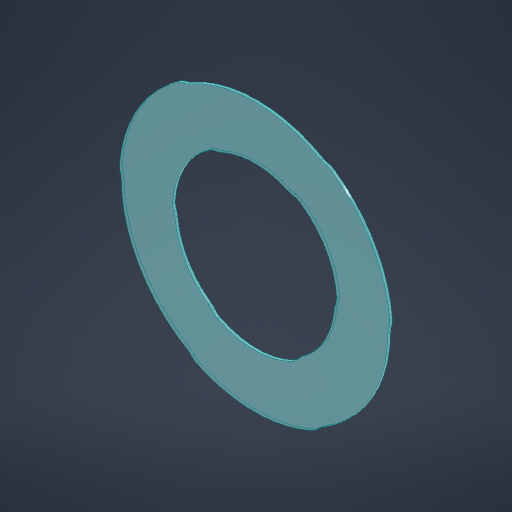
# Autodesk Inventor part: Lid_B
Saved by Autodesk Inventor 2026.1 (Build 301233020, 233B)
## iProperties
Created: 2023-08-16
Part Number: Lid_B
Material: PMMA Plastic
Document SubType Name: Modeling
Designer: Joshua Harper
Density: 1.188 g/cm^3
Appearance: Polycarbonate - Clear
Author: Joshua Harper
Autodesk Inventor part; units mm, degrees
ref_plane "YZ Plane" through (0, 0, 0) normal (1, 0, 0) x (0, 1, 0)
ref_plane "XZ Plane" through (0, 0, 0) normal (0, 1, 0) x (-1, 0, 0)
ref_plane "XY Plane" through (0, 0, 0) normal (0, 0, 1) x (1, 0, 0)
sketch "Sketch1" plane through (0, 0, 0) normal (0, 0, 1) x (1, 0, 0)
  circle A0 centre (0, 0) radius 106
  circle A1 centre (0, 0) radius 62.5
  dimension "d0" = 212
  dimension "d1" = 125
  constraints: 2 centre point, 2 coincident
  measures "d0" diameter of A0
  measures "d1" diameter of A1
extrude "Extrusion1" add sketch "Sketch1" along normal blind 2
sketch "Sketch2" plane through (0, 0, 0) normal (1, 0, 0) x (0, 1, 0)
  line L0 (106, 0) -> (-106, 0) projected
  line L1 (106, 0) -> (104.25, 0)
  line L2 (104.25, 0) -> (104.25, 2)
  line L3 (104.25, 2) -> (106, 2)
  line L4 (106, 2) -> (106, 0)
  line L5 (-62.5, 2) -> (-62.5, 0) projected
  line L6 (-62.5, 2) -> (-64.25, 2)
  line L7 (-64.25, 2) -> (-64.25, 0)
  line L8 (-64.25, 0) -> (-62.5, 0)
  line L9 (-62.5, 0) -> (-62.5, 2)
  line L10 (0, -0.4) -> (0, 2.4) projected
  point P0 (0, 0)
  dimension "d4" = 2
  dimension "d5" = 1.75
  dimension "d6" = 1.75
  dimension "d7" = 2
  constraints: 16 end point, 4 parallel, 2 horizontal, 2 perpendicular, 2 point on line
  measures "d4" distance of L1.end L2.end
  measures "d5" distance of L2.end L3.end
  measures "d6" distance between parallel lines of L7 L5
  measures "d7" distance between parallel lines of L6 L0
revolve "Revolution1" cut sketch "Sketch2" angle 66 mid plane about axis through (0, 0, -10) along (0, 0, 1)
fillet "Fillet1" radius 12 8 edges at (-56.7786, 87.4314, 1) (-57.7317, 88.8991, 1) (57.7317, 88.8991, 1) (56.7786, 87.4314, 1) (34.9931, -53.8846, 1) (34.0399, -52.4169, 1) (-34.9931, -53.8846, 1) (-34.0399, -52.4169, 1)
pattern_circular "Circular Pattern1" count 3 over 360 about axis through (0, 0, 0) along (0, 0, 1) of "Revolution1", "Fillet1"
body "Solid1"
